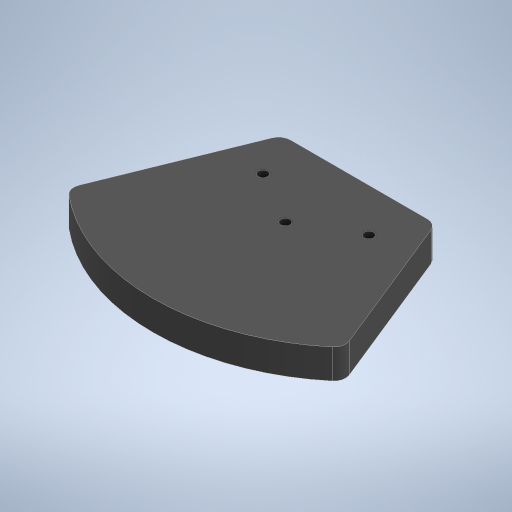
# Autodesk Inventor part: toe_sole_front_test
Saved by Autodesk Inventor 2024.1 (Build 281209000, 209)
## iProperties
Created: 2024-02-12
Part Number: toe_sole_front_test
Material: 一般
Document SubType Name: Modeling
Designer: hibik
Density: 1 g/cm^3
Appearance: 既定
Author: hibik
Autodesk Inventor part; units mm, degrees
ref_plane "YZ Plane" through (0, 0, 0) normal (1, 0, 0) x (0, 1, 0)
ref_plane "XZ Plane" through (0, 0, 0) normal (0, 1, 0) x (-1, 0, 0)
ref_plane "XY Plane" through (0, 0, 0) normal (0, 0, 1) x (1, 0, 0)
sketch "スケッチ1" plane through (0, 0, 0) normal (0, 1, 0) x (-1, 0, 0)
  line L0 (26, 0) -> (0, 0)
  line L1 (0, 0) -> (0, -15)
  line L2 (0, -15) -> (26, -15)
  line L3 (26, -15) -> (26, 0)
  line L4 (36.4849, 5.9511) -> (26, -20)
  line L5 (26, -20) -> (0, -20)
  line L6 (0, -20) -> (-10.4849, 5.9511)
  arc A0 (36.4849, 5.9511) -> (-10.4849, 5.9511) centre (13, -20) ccw
  line L7 (0, 0) -> (26, -15)
  line L8 (0, -15) -> (26, 0)
  line L9 (4, -2.3077) -> (22, -2.3077)
  line L10 (22, -2.3077) -> (22, -12.6923)
  line L11 (22, -12.6923) -> (4, -12.6923)
  line L12 (4, -12.6923) -> (4, -2.3077)
  circle A1 centre (4, -2.3077) radius 0.8
  circle A2 centre (4, -12.6923) radius 0.8
  circle A3 centre (22, -2.3077) radius 0.8
  circle A4 centre (22, -12.6923) radius 0.8
  circle A5 centre (13, -7.5) radius 0.8
  point P0 (22.6929, -13.0921)
  point P1 (21.2, -12.6923)
  dimension "d0" = 26
  dimension "d1" = 15
  dimension "d4" = 22
  dimension "d5" = 22
  dimension "d6" = 5
  dimension "d7" = 35
  dimension "d23" = 4
  dimension "d24" = 1.6
  dimension "d25" = 1.6
  dimension "d26" = 1.6
  dimension "d27" = 1.6
  dimension "d32" = 1.6
  constraints: 26 end point, 6 centre point, 6 coincident, 5 point on line, 4 parallel, 3 horizontal, 2 midpoint, 2 perpendicular, 2 point on circle
  measures "d0" distance of L0.start L0.end
  measures "d1" distance of L2.end L0.start
  measures "d4" angle of L3 L4
  measures "d5" angle of L6 L1
  measures "d6" distance between parallel lines of L5 L2
  measures "d7" radius of A0
  measures "d23" distance between parallel lines of L1 L12
  measures "d24" diameter of A1
  measures "d25" diameter of A2
  measures "d26" diameter of A3
  measures "d27" diameter of A4
  measures "d32" diameter of A5
extrude "押し出し1" add sketch "スケッチ1" along normal blind 4 contours L8 A3 L9 A1 L7 L0 | L3 L7 A4 L10 A3 L8 | L7 A1 L12 A2 L8 L1 | L2 L8 A2 L11 A4 L7 | A3 L10 L8 | L8 L9 A3 | A1 L9 L7 | L7 L12 A1 | L10 A3 L8 | L8 A3 L9 | A3 L8 A5 L7 A1 L9 | L9 A1 L7 | L7 A1 L12 | A1 L7 A5 L8 A2 L12 | L11 A2 L8 A5 L7 A4 | A3 L10 A4 L7 A5 L8 | L4 L5 L6 A0
sketch "スケッチ2" plane through (0, 0, 0) normal (0, -1, 0) x (1, 0, 0)
  arc A0 (-29.9016, 8.3432) -> (-34.0957, 5.3766) centre (-13, -20) ccw
  arc A1 (10.4849, 5.9511) -> (-36.4849, 5.9511) centre (-13, -20) ccw projected
  arc A2 (8.0957, 5.3766) -> (3.9016, 8.3432) centre (-13, -20) ccw
  line L0 (8.0957, 5.3766) -> (-1.349, -18)
  line L1 (-29.9016, 8.3432) -> (-19.2583, -18)
  line L2 (-34.0957, 5.3766) -> (-24.651, -18)
  line L3 (10.4849, 5.9511) -> (0, -20) projected
  line L4 (-26, -20) -> (-36.4849, 5.9511) projected
  line L5 (3.9016, 8.3432) -> (-6.7417, -18)
  line L6 (-24.651, -18) -> (-19.2583, -18)
  line L7 (0, -20) -> (-26, -20) projected
  line L8 (-6.7417, -18) -> (-1.349, -18)
  circle A3 centre (-4, -12.6923) radius 0.8 projected
  circle A4 centre (-22, -12.6923) radius 0.8 projected
  circle A5 centre (-4, -12.6923) radius 2.5
  circle A6 centre (-22, -12.6923) radius 2.5
  circle A7 centre (-13, -7.5) radius 0.8 projected
  circle A8 centre (-13, -7.5) radius 2.5
  arc A9 (-22.5806, 11.5787) -> (-29.9016, 8.3432) centre (-13, -20) ccw
  arc A10 (3.9016, 8.3432) -> (-3.4194, 11.5787) centre (-13, -20) ccw
  line L9 (-22.5806, 11.5787) -> (-19.3484, 3.5787)
  line L10 (-19.3484, 3.5787) -> (-26.7659, 0.5818)
  line L11 (-3.4194, 11.5787) -> (-6.6516, 3.5787)
  line L12 (-6.6516, 3.5787) -> (0.7659, 0.5818)
  point P0 (-22.3998, -10.2245)
  point P1 (-20.5733, -14.7452)
  point P2 (-5.4267, -14.7452)
  point P3 (-3.6002, -10.2245)
  dimension "d10" = 2
  dimension "d11" = 2
  dimension "d14" = 2
  dimension "d15" = 2
  dimension "d16" = 5
  dimension "d17" = 2
  dimension "d18" = 2
  dimension "d19" = 5
  dimension "d29" = 5
  dimension "d30" = 5
  dimension "d33" = 5
  dimension "d50" = 8
  dimension "d51" = 8
  dimension "d52" = 8
  dimension "d53" = 8
  constraints: 20 end point, 8 point on circle, 7 centre point, 6 concentric, 6 parallel, 4 perpendicular, 3 coincident, 2 point on line
  measures "d10" distance between parallel lines of L3 L0
  measures "d11" radial gap between concentric circles of A1 A2
  measures "d14" distance between parallel lines of L4 L2
  measures "d15" radial gap between concentric circles of A1 A0
  measures "d16" distance between parallel lines of L2 L1
  measures "d17" distance between parallel lines of L7 L6
  measures "d18" distance between parallel lines of L7 L8
  measures "d19" distance between parallel lines of L0 L5
  measures "d29" diameter of A5
  measures "d30" diameter of A6
  measures "d33" diameter of A8
  measures "d50" distance between parallel lines of L1 L9
  measures "d51" distance between parallel lines of L5 L11
  measures "d52" vertical distance of L11.start L11.end
  measures "d53" vertical distance of L9.start L9.end
extrude "押し出し2" add sketch "スケッチ2" along normal blind 1 contours L3 L7 L4 A1
fillet "フィレット1" radius 0.5 14 edges at (3.3734, -1, -6.3117) (2.6485, -1, 9.0538) (-6.0842, -1, -16.3726) (-1.4172, -1, -4.8213) (-4.0454, -1, -18) (-19.9158, -1, -16.3726) (-24.5828, -1, -4.8213) (-21.9546, -1, -18) (-29.3734, -1, -6.3117) (-28.6485, -1, 9.0538) (-5.0355, -1, 7.5787) (-2.9429, -1, 2.0802) (-20.9645, -1, 7.5787) (-23.0571, -1, 2.0802)
extrude "押し出し3" cut sketch "スケッチ2" against normal blind 1 contours A6 L1 A4 | L1 A4 A6 | A4 L1 | L1 A4 | A5 L5 A3 | L5 A3 A5 | A3 L5 | L5 A3 | A8
fillet "フィレット2" radius 2 4 edges at (10.4849, 1.5, 5.9511) (0, 1.5, -20) (-26, 1.5, -20) (-36.4849, 1.5, 5.9511)
equation "\"d5\" = d4"
